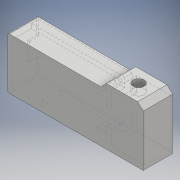
# Autodesk Inventor part: ttgo_lora_oled_case
Saved by Autodesk Inventor 2017 (Build 210142000, 142)
## iProperties
Created: 2021-11-16
Part Number: ttgo_lora_oled_case
Material: Generic
Document SubType Name: Modeling
Designer: simulator
Density: 1 g/cm^3
Appearance: Default
Author: simulator
## iProperties of the stored document ttgo_lora_oled_case_3DPrint.ipt
Created: 2021-11-16
Part Number: ttgo_lora_oled_case_3DPrint
Material: Generic
Document SubType Name: Modeling
Designer: simulator
Density: 1 g/cm^3
Appearance: Default
Author: simulator
Autodesk Inventor part; units mm, degrees
ref_plane "YZ Plane" through (0, 0, 0) normal (1, 0, 0) x (0, 1, 0)
ref_plane "XZ Plane" through (0, 0, 0) normal (0, 1, 0) x (-1, 0, 0)
ref_plane "XY Plane" through (0, 0, 0) normal (0, 0, 1) x (1, 0, 0)
sketch "Sketch1" plane through (0, 0, 0) normal (0, 1, 0) x (-1, 0, 0)
  line L0 (52, -10) -> (52, 16)
  arc A0 (52, 16) -> (51, 17) centre (51, 16) ccw
  line L1 (51, 17) -> (-22, 17)
  arc A1 (50, -10) -> (51, -9) centre (51, -10) ccw
  line L2 (-22, 17) -> (-22, -11)
  line L3 (-2, 20) -> (-19, 20)
  line L4 (-1, 5) -> (-1, 14)
  line L5 (0, 14) -> (0, 5)
  line L6 (-1, 1) -> (-1, -8)
  line L7 (51, 16) -> (-21, 16)
  line L8 (51, -2) -> (51, 8)
  line L9 (52, 8) -> (52, -2)
  line L10 (51, -10) -> (-21, -10)
  line L11 (51, 8) -> (52, 8)
  line L12 (52, 8) -> (52, -2)
  line L13 (52, -2) -> (51, -2)
  line L14 (51, -2) -> (51, 8)
  line L15 (51, -10) -> (51, 16)
  line L16 (52, 16) -> (52, -10)
  line L17 (51, -11) -> (-22, -11)
  line L18 (-21, 16) -> (-21, -10)
  line L19 (-2, 20) -> (1, 17)
  line L20 (-2, 20) -> (2.6568, 20) construction
  line L21 (-22, 17) -> (-19, 20)
  line L22 (-22, 17) -> (-5.0328, 17) construction
  line L23 (-1, 1) -> (0.3284, 1)
  line L24 (0.3284, 1) -> (0.3284, -8)
  line L25 (0.3284, -8) -> (-1, -8)
  line L26 (-1, -8) -> (-1, 1)
  line L27 (-1, 14) -> (0, 14)
  line L28 (0, 14) -> (0, 5)
  line L29 (0, 5) -> (-1, 5)
  line L30 (-1, 5) -> (-1, 14)
  point P0 (0, 0)
  dimension "d0" = 45
  dimension "d1" = 45
  constraints: 62 end point, 8 parallel, 6 point on circle, 5 horizontal, 4 perpendicular, 4 point on line, 2 centre point, 1 tangent
  measures "d0" angle of L19 L20
  measures "d1" angle of L22 L21
extrude "Extrusion1" add sketch "Sketch1" against normal blind 2 contours A1 L15 L13 L0 | A1 L10 L15 | L13 L8 L11 L0 | L17 L2 L1 A0 L0 L11 L15 L7 L18 L10 A1 | L15 L10 L18 L7 L8 | L21 L3 L19 L1 | L4 L27 L5 L29 | L23 L24 L25 L6
extrude "Extrusion2" add sketch "Sketch1" along normal blind 9 contours A1 L15 L13 L0 | A1 L10 L15 | L13 L8 L11 L0 | L17 L2 L1 A0 L0 L11 L15 L7 L18 L10 A1 | L21 L3 L19 L1
extrude "Extrusion3" add sketch "Sketch1" along normal blind 14 contours A1 L15 L13 L0 | A1 L10 L15 | L17 L2 L1 A0 L0 L11 L15 L7 L18 L10 A1 | L21 L3 L19 L1
sketch "Sketch2" plane through (0, 0, 0) normal (0, 1, 0) x (1, 0, 0)
  line L0 (-51, 10) -> (21, 10) projected
  line L1 (21, -16) -> (-51, -16) projected
  line L2 (21, 10) -> (-51, 10) projected
  line L3 (0, -16) -> (-5, -16)
  line L4 (-5, -16) -> (-5, -11)
  line L5 (-5, -11) -> (0, -11)
  line L6 (0, -11) -> (0, -16)
  line L7 (0, 10) -> (-5, 10)
  line L8 (-5, 10) -> (-5, 5)
  line L9 (-5, 5) -> (0, 5)
  line L10 (0, 5) -> (0, 10)
  line L11 (-5, 10) -> (-35, 10)
  line L12 (-35, 10) -> (-35, 7.5)
  line L13 (-35, 7.5) -> (-5, 7.5)
  line L14 (-5, 7.5) -> (-5, 10)
  line L15 (-51, 2) -> (-51, 10) projected
  line L16 (-5, -13.5) -> (-51, -13.5)
  line L17 (-51, -13.5) -> (-51, -16)
  line L18 (-51, -16) -> (-5, -16)
  line L19 (-5, -16) -> (-5, -13.5)
  point P0 (0, 0)
  dimension "d8" = 5
  dimension "d9" = 5
  dimension "d10" = 5
  dimension "d11" = 5
  dimension "d12" = 16
  constraints: 32 end point, 8 parallel, 4 horizontal, 4 perpendicular, 2 point on line, 1 midpoint
  measures "d8" distance of L4.end L5.end
  measures "d9" distance of L3.end L4.end
  measures "d10" distance of L9.end L8.end
  measures "d11" distance of L8.end L7.end
  measures "d12" distance between parallel lines of L12 L15
extrude "Extrusion4" add sketch "Sketch2" along normal blind 10
sketch "Sketch3" plane through (2, -2, 20) normal (0, 0, 1) x (1, 0, 0)
  line L0 (17, 0) -> (17, 16) projected
  line L1 (0, 16) -> (17, 2)
  circle A0 centre (8.5, 9) radius 3
  point P0 (-2, 2)
  dimension "d15" = 6
  constraints: 2 end point, 1 centre point, 1 midpoint, 1 point on line
  measures "d15" diameter of A0
sketch "Sketch4" plane through (0, 0, 0) normal (0, 1, 0) x (1, 0, 0)
  line L0 (0, -16) -> (21, -16) projected
  line L1 (-51, 10) -> (21, 10) projected
  line L2 (0, -16) -> (2.5, -16)
  line L3 (2.5, -16) -> (2.5, 10)
  line L4 (2.5, 10) -> (0, 10)
  line L5 (0, 10) -> (0, -16)
  line L6 (2.5, -8) -> (0, -8)
  line L7 (0, -8) -> (0, 2)
  line L8 (0, 2) -> (2.5, 2)
  line L9 (2.5, 2) -> (2.5, -8)
  line L10 (2.5, 2) -> (0, 2)
  line L11 (0, 2) -> (0, 10)
  line L12 (0, 10) -> (2.5, 10)
  line L13 (2.5, 10) -> (2.5, 2)
  line L14 (0, -8) -> (2.5, -8)
  line L15 (2.5, -8) -> (2.5, -16)
  line L16 (2.5, -16) -> (0, -16)
  line L17 (0, -16) -> (0, -8)
  point P0 (0, 0)
  dimension "d16" = 2.5
  dimension "d17" = 8
  dimension "d18" = 8
  constraints: 32 end point, 8 parallel, 4 horizontal, 4 perpendicular, 3 point on line
  measures "d16" distance of L4.end L3.end
  measures "d17" distance between parallel lines of L6 L0
  measures "d18" distance between parallel lines of L8 L1
extrude "Extrusion5" add sketch "Sketch4" along normal blind 14 contours L5 L6 L3 L0 | L5 L1 L3 L8
extrude "Extrusion6" cut sketch "Sketch3" against normal blind 14
sketch "Sketch5" plane through (0, 10, 0) normal (0, 1, 0) x (1, 0, 0)
  line L0 (-35, 10) -> (0, 10) projected
  line L1 (-35, 10) -> (-35, 7.5) projected
  line L2 (-35, 7.5) -> (-5, 7.5) projected
  line L3 (-5, 7.5) -> (-5, 5) projected
  line L4 (-5, 5) -> (0, 5) projected
  line L5 (0, 5) -> (0, 10) projected
  line L6 (0, -16) -> (-51, -16) projected
  line L7 (0, -16) -> (0, -11) projected
  line L8 (0, -11) -> (-5, -11) projected
  line L9 (-5, -11) -> (-5, -13.5) projected
  line L10 (-5, -13.5) -> (-51, -13.5) projected
  line L11 (-51, -16) -> (-51, -13.5) projected
  line L12 (-5, -11) -> (0, -16)
  line L13 (0, 5) -> (0, 10) projected
  line L14 (0, 10) -> (-5, 5)
  point P0 (0, 0)
  point P1 (-2.5, 7.5)
  point P2 (-2.5, -13.5)
  constraints: 4 end point, 2 midpoint
hole "Hole1" at (-2.5, 10, -7.5) at (-2.5, 10, 13.5) direction (0, -1, 0) diameter 2 depth 8 tip angle 118
body "Solid1"
